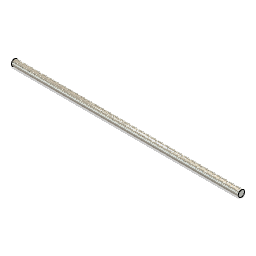
final assembly v7 (Autodesk Fusion 360 archive; units mm, degrees)
design "rod3"
Autodesk Fusion 360 part; units mm, degrees
sketch "Sketch1" plane through (0, 0, 0) normal (1, 0, 0) x (0, 0, -1)
  circle A0 centre (0, 0) radius 3
  dimension "d1" = 6
  constraint coincident A0.centre origin
  measures "d1" diameter of A0
extrude "Extrude1" add sketch "Sketch1" along normal blind 215

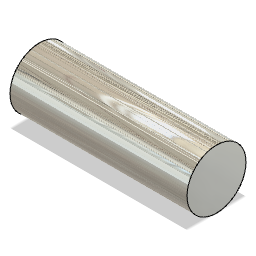
design "rod4"
Autodesk Fusion 360 part; units mm, degrees
sketch "Sketch1" plane through (0, 0, 0) normal (1, 0, 0) x (0, 0, -1)
  circle A0 centre (0, 0) radius 3
  dimension "d1" = 6
  constraint coincident A0.centre origin
  measures "d1" diameter of A0
extrude "Extrude1" add sketch "Sketch1" along normal blind 18

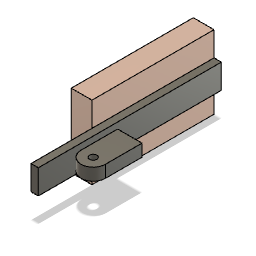
design "stamp pad 1"
Autodesk Fusion 360 part; units mm, degrees
sketch "Sketch1" plane through (0, 0, 0) normal (1, 0, 0) x (0, 0, -1)
  line L0 (-50, 30) -> (50, 30)
  line L1 (50, 30) -> (50, -30)
  line L2 (50, -30) -> (-50, -30)
  line L3 (-50, -30) -> (-50, 30)
  line L4 (48, -28) -> (-48, -28)
  line L5 (-48, -28) -> (-48, 28)
  line L6 (-48, 28) -> (48, 28)
  line L7 (48, 28) -> (48, -28)
  dimension "d1" = 100
  dimension "d2" = 60
  dimension "d3" = 2
  dimension "d17" = 30
  dimension "d18" = 50
  constraint horizontal L0
  constraint perpendicular L0 L1
  constraint parallel L0 L2
  constraint parallel L1 L3
  measures "d1" distance of L1.end L2.end
  measures "d2" distance of L0.end L1.end
  measures "d17" distance of L0 origin
  measures "d18" distance of origin L3
extrude "Extrude1" add sketch "Sketch1" along normal blind 2 contours L0 L1 L2 L3 | L4 L5 L6 L7 makes body 1
extrude "Extrude2" add sketch "Sketch1" against normal blind 15 bodies 1
sketch "Sketch2" plane through (0, 0, 0) normal (-1, 0, 0) x (0, 0, 1)
  line L0 (-48, 28) -> (-48, -28)
  line L1 (-48, -28) -> (48, -28)
  line L2 (48, -28) -> (48, 28)
  line L3 (48, 28) -> (-48, 28)
  line L4 (45, 25) -> (-45, 25)
  line L5 (-45, 25) -> (-45, -25)
  line L6 (-45, -25) -> (45, -25)
  line L7 (45, -25) -> (45, 25)
  line L8 (45, 25) -> (-45, -25) construction
  line L9 (-45, 25) -> (45, -25) construction
  dimension "d8" = 90
  dimension "d9" = 50
  constraint horizontal L4
  constraint perpendicular L4 L5
  constraint parallel L4 L6
  constraint parallel L5 L7
  constraint coincident L8 origin
  constraint coincident L9 origin
  measures "d8" distance of L5.end L6.end
  measures "d9" distance of L4.end L5.end
extrude "Extrude3" add sketch "Sketch2" along normal blind 13 contours L4 L5 L6 L7 bodies 1
sketch "Sketch4" plane through (2, 0, 0) normal (1, 0, 0) x (0, 0, -1)
  line L0 (-50, -30) -> (50, -30)
  line L1 (50, -30) -> (50, 30)
  line L2 (50, 30) -> (-50, 30)
  line L3 (-50, 30) -> (-50, -30)
  line L4 (50, -10) -> (-100, -10)
  line L5 (-100, -10) -> (-100, 10)
  line L6 (-100, 10) -> (50, 10)
  line L7 (50, 10) -> (50, -10)
  point P0 (-50, -10)
  point P1 (50, -10)
  dimension "d22" = 20
  constraint coincident L3 P0
  constraint horizontal L4
  constraint vertical L5
  constraint horizontal L6
  constraint vertical L7
  constraint coincident P1 L4.start
  measures "d22" distance of P1 L6.end
extrude "Extrude4" add sketch "Sketch4" along normal blind 6 contours L3 L4 L5 L6 | L1 L3 L4 L6 L7 bodies 1
sketch "Sketch5" plane through (0, -10, 0) normal (0, -1, 0) x (1, 0, 0)
  line L0 (2, 50) -> (2, -50)
  line L1 (2, -50) -> (8, -50)
  line L2 (8, -50) -> (8, 100)
  line L3 (8, 100) -> (2, 100)
  line L4 (2, 100) -> (2, 50)
  circle A0 centre (18, 65) radius 3
  line L5 (28, 65) -> (28, 35)
  line L6 (28, 35) -> (8, 35)
  arc A1 (28, 65) -> (8, 65) centre (18, 65) ccw
  dimension "d26" = 10
  dimension "d27" = 6
  constraint coincident L2 A1.end
  constraint concentric A0 A1
  constraint tangent L5 A1
  constraint parallel L2 L5
  constraint coincident L2 L6.end
  constraint perpendicular L2 L6
  measures "d26" distance of A1.end A0.centre
  measures "d27" diameter of A0
extrude "Extrude5" add sketch "Sketch5" against normal blind 10 from surface at -5 contours L2 L5 L6 A1 bodies 1
sketch "Sketch6" plane through (0, -30, 0) normal (0, -1, 0) x (1, 0, 0)
  line L0 (-15, -50) -> (2, -50)
  line L1 (2, -50) -> (2, 50)
  line L2 (2, 50) -> (-15, 50)
  line L3 (-15, 50) -> (-15, -50)
  line L4 (-3.4442, -44.9299) -> (-3.4442, 44.3486) construction
  line L5 (-3.4442, 44.3486) -> (-9.7091, 44.3486) construction
  line L6 (-9.7091, 44.3486) -> (-9.7091, -44.9299) construction
  line L7 (-9.7091, -44.9299) -> (-3.4442, -44.9299) construction
  dimension "d32" = 10
  text T0 "STAMP PAD" font "Arial" height 10 align centre middle in box 89.2785 x 6.2649 at (-3.4442, -44.9299) x (0, 1) y (-1, 0) spacing 1 kerned
emboss "Emboss2" depth -2 profiles "Sketch6" section 1 text T0 onto face at (-9.3333, -30, -16.6667) on bodies 1 bodies 1 makes body 2 at (-8.0137, -28, 2.4504) makes body 3 at (-6.6062, -30, 24.3399) makes body 4 at (-8.0137, -30, 15.3972) makes body 5 at (-6.6017, -28, 34.5536) makes body 6 at (-6.6062, -28, -17.8429)

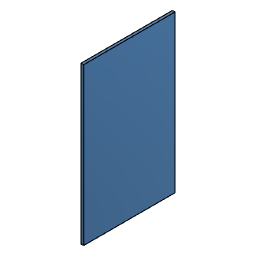
design "base"
Autodesk Fusion 360 part; units mm, degrees
sketch "Sketch1" plane through (0, 0, 0) normal (1, 0, 0) x (0, 0, -1)
  line L0 (0, 0) -> (-350, 0)
  line L1 (-350, 0) -> (-350, 600)
  line L2 (-350, 600) -> (0, 600)
  line L3 (0, 600) -> (0, 0)
  dimension "d1" = 350
  dimension "d2" = 600
  constraint horizontal L0
  constraint vertical L1
  constraint horizontal L2
  constraint vertical L3
  constraint coincident L0.start L3.end
  measures "d1" distance of L0.start L0.end
  measures "d2" distance of L0.start L2.end
extrude "Extrude1" add sketch "Sketch1" along normal blind 10

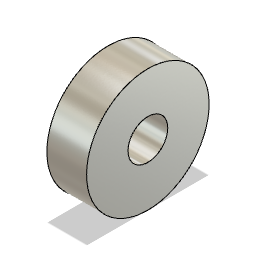
design "bearings"
Autodesk Fusion 360 part; units mm, degrees
sketch "Sketch1" plane through (0, 0, 0) normal (1, 0, 0) x (0, 0, -1)
  circle A0 centre (0, 0) radius 3
  circle A1 centre (0, 0) radius 9.25
  dimension "d1" = 6
  dimension "d2" = 18.5
  constraint coincident A0.centre A1.centre
  constraint concentric A0 A1
  measures "d1" diameter of A0
  measures "d2" diameter of A1
extrude "Extrude1" add sketch "Sketch1" along normal blind 6

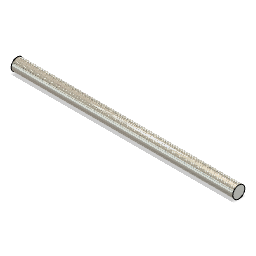
design "rod1"
Autodesk Fusion 360 part; units mm, degrees
sketch "Sketch1" plane through (0, 0, 0) normal (1, 0, 0) x (0, 0, -1)
  circle A0 centre (0, 0) radius 3
  dimension "d1" = 6
  constraint coincident A0.centre origin
  measures "d1" diameter of A0
extrude "Extrude1" add sketch "Sketch1" along normal blind 110

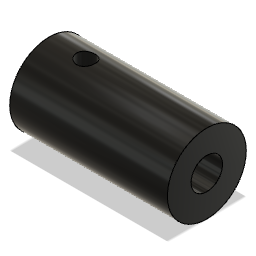
design "motor connector v2"
Autodesk Fusion 360 part; units mm, degrees
sketch "Sketch1" plane through (0, 0, 0) normal (1, 0, 0) x (0, 0, -1)
  circle A0 centre (0, 0) radius 3
  circle A1 centre (0, 0) radius 7.5
  dimension "d1" = 6
  dimension "d2" = 15
  constraint coincident A0.centre A1.centre
  measures "d1" diameter of A0
  measures "d2" diameter of A1
extrude "Extrude1" add sketch "Sketch1" against normal blind 15
sketch "Sketch2" plane through (-15, 0, 0) normal (-1, 0, 0) x (0, 0, 1)
  circle A0 centre (0, 0) radius 7.5
  circle A1 centre (0, 0) radius 3.25
  circle A2 centre (0, 0) radius 7.5
  dimension "d5" = 6.5
  constraint concentric A1 A2
  measures "d5" diameter of A1
extrude "Extrude2" add sketch "Sketch2" along normal blind 15
sketch "Sketch3" plane through (0, 0, 0) normal (0, 1, 0) x (1, 0, 0)
  line L0 (-30, 7.5) -> (-30, -7.5)
  line L1 (0, -7.5) -> (0, 7.5)
  circle A0 centre (-23, 0) radius 1.75
  point P0 (-23, 0)
  dimension "d8" = 30
  constraint coincident P0 A0.centre
  measures "d8" distance of L0 L1
extrude "Extrude3" cut sketch "Sketch3" along normal mid plane 38

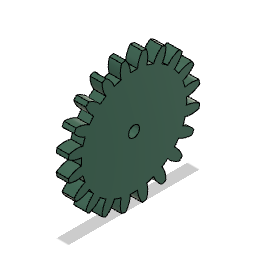
design "6 cm gear"
Autodesk Fusion 360 part; units mm, degrees
sketch "Sketch1" plane through (0, 0, 0) normal (1, 0, 0) x (0, 0, -1)
  arc A0 (28.2536, 4.8202) -> (28.2536, 8.3351) centre (2.0635, 6.5776) ccw
  arc A1 (28.2536, 8.3351) -> (34.8066, 10.6867) centre (27.6511, 20.3199) ccw
  arc A2 (17.9851, 35.4827) -> (16.0896, 36.4485) centre (2.0635, 6.5776) ccw
  arc A3 (8.4852, 32.029) -> (8.2737, 38.988) centre (-3.0992, 35.1595) ccw
  arc A4 (34.8066, 10.6867) -> (34.4738, 12.7878) centre (2.0635, 6.5776) ccw
  arc A5 (6.1726, 39.3208) -> (3.8209, 32.7677) centre (15.8058, 32.1653) ccw
  arc A6 (18.8794, -13.5776) -> (24.6337, -17.4969) centre (28.2213, -6.0457) ccw
  arc A7 (16.0896, -23.2932) -> (17.9851, -22.3274) centre (2.0635, 6.5776) ccw
  arc A8 (22.2187, -10.2383) -> (24.2847, -7.3947) centre (2.0635, 6.5776) ccw
  arc A9 (3.8209, 32.7677) -> (0.306, 32.7677) centre (2.0635, 6.5776) ccw
  arc A10 (0.306, -19.6125) -> (3.8209, -19.6125) centre (2.0635, 6.5776) ccw
  arc A11 (24.6337, -17.4969) -> (26.138, -15.9926) centre (2.0635, 6.5776) ccw
  arc A12 (-13.8582, -22.3274) -> (-11.9627, -23.2932) centre (2.0635, 6.5776) ccw
  arc A13 (31.9343, -7.4485) -> (26.4286, -3.187) centre (22.1521, -14.3991) ccw
  arc A14 (6.1726, 39.3208) -> (3.8209, 32.7677) centre (15.8058, 32.1653) ccw
  arc A15 (-14.7525, -13.5776) -> (-11.9089, -15.6436) centre (2.0635, 6.5776) ccw
  arc A16 (8.2737, -25.8327) -> (8.4852, -18.8737) centre (-3.0992, -22.0043) ccw
  arc A17 (-7.7012, -17.7875) -> (-4.3583, -18.8737) centre (2.0635, 6.5776) ccw
  arc A18 (0.306, -19.6125) -> (3.8209, -19.6125) centre (2.0635, 6.5776) ccw
  arc A19 (26.4286, -3.187) -> (27.5148, 0.1559) centre (2.0635, 6.5776) ccw
  arc A20 (8.4852, -18.8737) -> (11.8281, -17.7875) centre (2.0635, 6.5776) ccw
  arc A21 (8.2737, 38.988) -> (6.1726, 39.3208) centre (2.0635, 6.5776) ccw
  arc A22 (6.1726, -26.1655) -> (8.2737, -25.8327) centre (2.0635, 6.5776) ccw
  arc A23 (8.4852, -18.8737) -> (11.8281, -17.7875) centre (2.0635, 6.5776) ccw
  arc A24 (11.8281, -17.7875) -> (16.0896, -23.2932) centre (23.0402, -13.5111) ccw
  arc A25 (30.9685, -9.344) -> (31.9343, -7.4485) centre (2.0635, 6.5776) ccw
  arc A26 (17.9851, -22.3274) -> (16.0358, -15.6436) centre (5.9857, -22.2007) ccw
  arc A27 (6.1726, -26.1655) -> (8.2737, -25.8327) centre (2.0635, 6.5776) ccw
  arc A28 (3.8209, -19.6125) -> (6.1726, -26.1655) centre (15.8058, -19.01) ccw
  arc A29 (34.4738, 0.3674) -> (34.8066, 2.4685) centre (2.0635, 6.5776) ccw
  arc A30 (34.8066, 2.4685) -> (28.2536, 4.8202) centre (27.6511, -7.1647) ccw
  arc A31 (18.8794, 26.7329) -> (16.0358, 28.7989) centre (2.0635, 6.5776) ccw
  arc A32 (-11.9089, -15.6436) -> (-13.8582, -22.3274) centre (-1.8588, -22.2007) ccw
  arc A33 (11.8281, -17.7875) -> (16.0896, -23.2932) centre (23.0402, -13.5111) ccw
  arc A34 (8.4852, 32.029) -> (8.2737, 38.988) centre (-3.0992, 35.1595) ccw
  arc A35 (16.0896, -23.2932) -> (17.9851, -22.3274) centre (2.0635, 6.5776) ccw
  arc A36 (16.0896, 36.4485) -> (11.8281, 30.9428) centre (23.0402, 26.6663) ccw
  arc A37 (16.0358, -15.6436) -> (18.8794, -13.5776) centre (2.0635, 6.5776) ccw
  arc A38 (-4.3583, -18.8737) -> (-4.1467, -25.8327) centre (7.2261, -22.0043) ccw
  arc A39 (-11.9627, -23.2932) -> (-7.7012, -17.7875) centre (-18.9133, -13.5111) ccw
  arc A40 (3.8209, -19.6125) -> (6.1726, -26.1655) centre (15.8058, -19.01) ccw
  arc A41 (11.8281, 30.9428) -> (8.4852, 32.029) centre (2.0635, 6.5776) ccw
  arc A42 (-4.1467, -25.8327) -> (-2.0457, -26.1655) centre (2.0635, 6.5776) ccw
  arc A43 (17.9851, -22.3274) -> (16.0358, -15.6436) centre (5.9857, -22.2007) ccw
  arc A44 (16.0358, -15.6436) -> (18.8794, -13.5776) centre (2.0635, 6.5776) ccw
  arc A45 (24.2847, -7.3947) -> (30.9685, -9.344) centre (30.8418, 2.6554) ccw
  arc A46 (30.9685, 22.4993) -> (24.2847, 20.55) centre (30.8418, 10.4999) ccw
  arc A47 (18.8794, 26.7329) -> (16.0358, 28.7989) centre (2.0635, 6.5776) ccw
  arc A48 (26.138, 29.1479) -> (24.6337, 30.6521) centre (2.0635, 6.5776) ccw
  arc A49 (24.2847, 20.55) -> (22.2187, 23.3936) centre (2.0635, 6.5776) ccw
  arc A50 (27.5148, 12.9994) -> (26.4286, 16.3423) centre (2.0635, 6.5776) ccw
  arc A51 (17.9851, 35.4827) -> (16.0896, 36.4485) centre (2.0635, 6.5776) ccw
  arc A52 (31.9343, 20.6038) -> (30.9685, 22.4993) centre (2.0635, 6.5776) ccw
  arc A53 (8.2737, 38.988) -> (6.1726, 39.3208) centre (2.0635, 6.5776) ccw
  arc A54 (16.0896, 36.4485) -> (11.8281, 30.9428) centre (23.0402, 26.6663) ccw
  arc A55 (24.6337, 30.6521) -> (18.8794, 26.7329) centre (28.2213, 19.201) ccw
  arc A56 (16.0358, 28.7989) -> (17.9851, 35.4827) centre (5.9857, 35.356) ccw
  arc A57 (-2.0457, -26.1655) -> (0.306, -19.6125) centre (-11.6789, -19.01) ccw
  arc A58 (16.0358, 28.7989) -> (17.9851, 35.4827) centre (5.9857, 35.356) ccw
  arc A59 (27.5148, 0.1559) -> (34.4738, 0.3674) centre (30.6454, 11.7403) ccw
  arc A60 (8.2737, -25.8327) -> (8.4852, -18.8737) centre (-3.0992, -22.0043) ccw
  arc A61 (3.8209, 32.7677) -> (0.306, 32.7677) centre (2.0635, 6.5776) ccw
  arc A62 (26.4286, 16.3423) -> (31.9343, 20.6038) centre (22.1521, 27.5544) ccw
  arc A63 (22.2187, 23.3936) -> (26.138, 29.1479) centre (14.6868, 32.7354) ccw
  arc A64 (11.8281, 30.9428) -> (8.4852, 32.029) centre (2.0635, 6.5776) ccw
  arc A65 (34.4738, 12.7878) -> (27.5148, 12.9994) centre (30.6454, 1.4149) ccw
  arc A66 (-27.8074, -7.4485) -> (-26.8416, -9.344) centre (2.0635, 6.5776) ccw
  arc A67 (30.9685, 22.4993) -> (24.2847, 20.55) centre (30.8418, 10.4999) ccw
  arc A68 (-14.7525, -13.5776) -> (-11.9089, -15.6436) centre (2.0635, 6.5776) ccw
  arc A69 (-7.7012, -17.7875) -> (-4.3583, -18.8737) centre (2.0635, 6.5776) ccw
  arc A70 (-4.3583, -18.8737) -> (-4.1467, -25.8327) centre (7.2261, -22.0043) ccw
  arc A71 (-20.5068, -17.4969) -> (-14.7525, -13.5776) centre (-24.0944, -6.0457) ccw
  arc A72 (-13.8582, -22.3274) -> (-11.9627, -23.2932) centre (2.0635, 6.5776) ccw
  arc A73 (-18.0918, -10.2383) -> (-22.0111, -15.9926) centre (-10.5599, -19.5802) ccw
  arc A74 (-30.6797, 2.4685) -> (-30.3469, 0.3674) centre (2.0635, 6.5776) ccw
  arc A75 (-27.8074, 20.6038) -> (-22.3017, 16.3423) centre (-18.0252, 27.5544) ccw
  arc A76 (-11.9089, 28.7989) -> (-14.7525, 26.7329) centre (2.0635, 6.5776) ccw
  arc A77 (24.6337, 30.6521) -> (18.8794, 26.7329) centre (28.2213, 19.201) ccw
  arc A78 (-18.0918, 23.3936) -> (-20.1578, 20.55) centre (2.0635, 6.5776) ccw
  arc A79 (-30.3469, 0.3674) -> (-23.3879, 0.1559) centre (-26.5185, 11.7403) ccw
  arc A80 (34.4738, 0.3674) -> (34.8066, 2.4685) centre (2.0635, 6.5776) ccw
  arc A81 (-7.7012, 30.9428) -> (-11.9627, 36.4485) centre (-18.9133, 26.6663) ccw
  arc A82 (34.8066, 2.4685) -> (28.2536, 4.8202) centre (27.6511, -7.1647) ccw
  arc A83 (-4.1467, 38.988) -> (-4.3583, 32.029) centre (7.2261, 35.1595) ccw
  arc A84 (-18.0918, -10.2383) -> (-22.0111, -15.9926) centre (-10.5599, -19.5802) ccw
  arc A85 (26.138, 29.1479) -> (24.6337, 30.6521) centre (2.0635, 6.5776) ccw
  arc A86 (-22.0111, -15.9926) -> (-20.5068, -17.4969) centre (2.0635, 6.5776) ccw
  arc A87 (-20.1578, -7.3947) -> (-18.0918, -10.2383) centre (2.0635, 6.5776) ccw
  arc A88 (-24.1266, 8.3351) -> (-24.1266, 4.8202) centre (2.0635, 6.5776) ccw
  arc A89 (-26.8416, -9.344) -> (-20.1578, -7.3947) centre (-26.7149, 2.6554) ccw
  arc A90 (22.2187, 23.3936) -> (26.138, 29.1479) centre (14.6868, 32.7354) ccw
  arc A91 (28.2536, 4.8202) -> (28.2536, 8.3351) centre (2.0635, 6.5776) ccw
  arc A92 (24.6337, -17.4969) -> (26.138, -15.9926) centre (2.0635, 6.5776) ccw
  arc A93 (-27.8074, -7.4485) -> (-26.8416, -9.344) centre (2.0635, 6.5776) ccw
  arc A94 (22.2187, -10.2383) -> (24.2847, -7.3947) centre (2.0635, 6.5776) ccw
  arc A95 (34.8066, 10.6867) -> (34.4738, 12.7878) centre (2.0635, 6.5776) ccw
  arc A96 (27.5148, 12.9994) -> (26.4286, 16.3423) centre (2.0635, 6.5776) ccw
  arc A97 (24.2847, 20.55) -> (22.2187, 23.3936) centre (2.0635, 6.5776) ccw
  arc A98 (28.2536, 8.3351) -> (34.8066, 10.6867) centre (27.6511, 20.3199) ccw
  arc A99 (-26.8416, 22.4993) -> (-27.8074, 20.6038) centre (2.0635, 6.5776) ccw
  arc A100 (-11.9627, -23.2932) -> (-7.7012, -17.7875) centre (-18.9133, -13.5111) ccw
  arc A101 (27.5148, 0.1559) -> (34.4738, 0.3674) centre (30.6454, 11.7403) ccw
  arc A102 (34.4738, 12.7878) -> (27.5148, 12.9994) centre (30.6454, 1.4149) ccw
  arc A103 (-22.3017, -3.187) -> (-27.8074, -7.4485) centre (-18.0252, -14.3991) ccw
  arc A104 (-20.5068, 30.6521) -> (-22.0111, 29.1479) centre (2.0635, 6.5776) ccw
  arc A105 (26.138, -15.9926) -> (22.2187, -10.2383) centre (14.6868, -19.5802) ccw
  arc A106 (26.4286, -3.187) -> (27.5148, 0.1559) centre (2.0635, 6.5776) ccw
  arc A107 (18.8794, -13.5776) -> (24.6337, -17.4969) centre (28.2213, -6.0457) ccw
  arc A108 (30.9685, -9.344) -> (31.9343, -7.4485) centre (2.0635, 6.5776) ccw
  arc A109 (31.9343, -7.4485) -> (26.4286, -3.187) centre (22.1521, -14.3991) ccw
  arc A110 (-23.3879, 0.1559) -> (-22.3017, -3.187) centre (2.0635, 6.5776) ccw
  arc A111 (26.4286, 16.3423) -> (31.9343, 20.6038) centre (22.1521, 27.5544) ccw
  arc A112 (31.9343, 20.6038) -> (30.9685, 22.4993) centre (2.0635, 6.5776) ccw
  arc A113 (-30.3469, 0.3674) -> (-23.3879, 0.1559) centre (-26.5185, 11.7403) ccw
  arc A114 (24.2847, -7.3947) -> (30.9685, -9.344) centre (30.8418, 2.6554) ccw
  arc A115 (-14.7525, 26.7329) -> (-20.5068, 30.6521) centre (-24.0944, 19.201) ccw
  arc A116 (-26.8416, -9.344) -> (-20.1578, -7.3947) centre (-26.7149, 2.6554) ccw
  arc A117 (-20.1578, -7.3947) -> (-18.0918, -10.2383) centre (2.0635, 6.5776) ccw
  arc A118 (0.306, 32.7677) -> (-2.0457, 39.3208) centre (-11.6789, 32.1653) ccw
  arc A119 (-24.1266, 4.8202) -> (-30.6797, 2.4685) centre (-23.5242, -7.1647) ccw
  arc A120 (-26.8416, 22.4993) -> (-27.8074, 20.6038) centre (2.0635, 6.5776) ccw
  arc A121 (-30.3469, 12.7878) -> (-30.6797, 10.6867) centre (2.0635, 6.5776) ccw
  arc A122 (-11.9089, -15.6436) -> (-13.8582, -22.3274) centre (-1.8588, -22.2007) ccw
  arc A123 (-4.1467, -25.8327) -> (-2.0457, -26.1655) centre (2.0635, 6.5776) ccw
  arc A124 (-23.3879, 12.9994) -> (-30.3469, 12.7878) centre (-26.5185, 1.4149) ccw
  arc A125 (-22.0111, 29.1479) -> (-18.0918, 23.3936) centre (-10.5599, 32.7354) ccw
  arc A126 (-22.3017, -3.187) -> (-27.8074, -7.4485) centre (-18.0252, -14.3991) ccw
  arc A127 (-20.5068, -17.4969) -> (-14.7525, -13.5776) centre (-24.0944, -6.0457) ccw
  arc A128 (-4.3583, 32.029) -> (-7.7012, 30.9428) centre (2.0635, 6.5776) ccw
  arc A129 (-2.0457, 39.3208) -> (-4.1467, 38.988) centre (2.0635, 6.5776) ccw
  arc A130 (-18.0918, 23.3936) -> (-20.1578, 20.55) centre (2.0635, 6.5776) ccw
  arc A131 (-23.3879, 0.1559) -> (-22.3017, -3.187) centre (2.0635, 6.5776) ccw
  arc A132 (-20.1578, 20.55) -> (-26.8416, 22.4993) centre (-26.7149, 10.4999) ccw
  arc A133 (-27.8074, 20.6038) -> (-22.3017, 16.3423) centre (-18.0252, 27.5544) ccw
  arc A134 (-2.0457, -26.1655) -> (0.306, -19.6125) centre (-11.6789, -19.01) ccw
  arc A135 (-22.0111, -15.9926) -> (-20.5068, -17.4969) centre (2.0635, 6.5776) ccw
  arc A136 (-24.1266, 8.3351) -> (-24.1266, 4.8202) centre (2.0635, 6.5776) ccw
  arc A137 (-24.1266, 4.8202) -> (-30.6797, 2.4685) centre (-23.5242, -7.1647) ccw
  arc A138 (-14.7525, 26.7329) -> (-20.5068, 30.6521) centre (-24.0944, 19.201) ccw
  arc A139 (-11.9627, 36.4485) -> (-13.8582, 35.4827) centre (2.0635, 6.5776) ccw
  arc A140 (-2.0457, 39.3208) -> (-4.1467, 38.988) centre (2.0635, 6.5776) ccw
  arc A141 (-20.1578, 20.55) -> (-26.8416, 22.4993) centre (-26.7149, 10.4999) ccw
  arc A142 (-30.3469, 12.7878) -> (-30.6797, 10.6867) centre (2.0635, 6.5776) ccw
  arc A143 (-20.5068, 30.6521) -> (-22.0111, 29.1479) centre (2.0635, 6.5776) ccw
  arc A144 (-4.1467, 38.988) -> (-4.3583, 32.029) centre (7.2261, 35.1595) ccw
  arc A145 (-11.9627, 36.4485) -> (-13.8582, 35.4827) centre (2.0635, 6.5776) ccw
  arc A146 (-30.6797, 2.4685) -> (-30.3469, 0.3674) centre (2.0635, 6.5776) ccw
  arc A147 (0.306, 32.7677) -> (-2.0457, 39.3208) centre (-11.6789, 32.1653) ccw
  arc A148 (-23.3879, 12.9994) -> (-30.3469, 12.7878) centre (-26.5185, 1.4149) ccw
  arc A149 (-13.8582, 35.4827) -> (-11.9089, 28.7989) centre (-1.8588, 35.356) ccw
  arc A150 (-13.8582, 35.4827) -> (-11.9089, 28.7989) centre (-1.8588, 35.356) ccw
  arc A151 (-22.3017, 16.3423) -> (-23.3879, 12.9994) centre (2.0635, 6.5776) ccw
  arc A152 (-4.3583, 32.029) -> (-7.7012, 30.9428) centre (2.0635, 6.5776) ccw
  arc A153 (-11.9089, 28.7989) -> (-14.7525, 26.7329) centre (2.0635, 6.5776) ccw
  arc A154 (-22.3017, 16.3423) -> (-23.3879, 12.9994) centre (2.0635, 6.5776) ccw
  arc A155 (-22.0111, 29.1479) -> (-18.0918, 23.3936) centre (-10.5599, 32.7354) ccw
  arc A156 (-7.7012, 30.9428) -> (-11.9627, 36.4485) centre (-18.9133, 26.6663) ccw
  arc A157 (-30.6797, 10.6867) -> (-24.1266, 8.3351) centre (-23.5242, 20.3199) ccw
  arc A158 (-30.6797, 10.6867) -> (-24.1266, 8.3351) centre (-23.5242, 20.3199) ccw
  arc A159 (26.138, -15.9926) -> (22.2187, -10.2383) centre (14.6868, -19.5802) ccw
  circle A160 centre (2.0635, 6.5776) radius 2.75
  dimension "d4" = 5.5
  constraint concentric A88 A160
  measures "d4" diameter of A160
extrude "Extrude1" add sketch "Sketch1" along normal blind 6

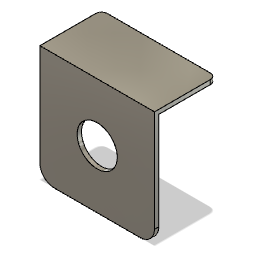
design "Motor clamp"
Autodesk Fusion 360 part; units mm, degrees
sketch "Sketch1" plane through (0, 0, 0) normal (0, 1, 0) x (1, 0, 0)
  line L0 (18, 10.75) -> (-18, 10.75)
  line L1 (-20, 8.75) -> (-20, -10.75)
  line L2 (-20, -10.75) -> (20, -10.75)
  line L3 (20, -10.75) -> (20, 8.75)
  line L4 (20, 10.75) -> (-20, -10.75) construction
  line L5 (-20, 10.75) -> (20, -10.75) construction
  arc A0 (-18, 10.75) -> (-20, 8.75) centre (-18, 8.75) ccw
  arc A1 (20, 8.75) -> (18, 10.75) centre (18, 8.75) ccw
  dimension "d1" = 40
  dimension "d2" = 21.5
  dimension "d3" = 2
  constraint horizontal L0
  constraint perpendicular L0 L1
  constraint parallel L0 L2
  constraint parallel L1 L3
  constraint coincident L4 origin
  constraint coincident L5 origin
  constraint coincident L5.start L0
  constraint coincident L5.start L1
  constraint tangent L0 A0
  constraint tangent L1 A0
  constraint coincident L4.start L0
  constraint coincident L4.start L3
  constraint tangent L0 A1
  constraint tangent L3 A1
  constraint equal A0 A1
  measures "d1" distance of L1.end L2.end
  measures "d2" distance of L5.start L1.end
  measures "d3" radius of A0
extrude "Extrude1" add sketch "Sketch1" along normal blind 1.5
sketch "Sketch2" plane through (0, 0, 10.75) normal (0, 0, 1) x (1, 0, 0)
  line L0 (-20, 0) -> (20, 0)
  line L1 (20, 0) -> (20, 1.5)
  line L2 (20, 1.5) -> (-20, 1.5)
  line L3 (-20, 1.5) -> (-20, 0)
  line L4 (-20, 1.5) -> (20, 1.5)
  line L5 (20, 1.5) -> (20, -34)
  line L6 (15, -39) -> (-15, -39)
  line L7 (-20, -34) -> (-20, 1.5)
  circle A0 centre (0, -18.75) radius 7
  arc A1 (-20, -34) -> (-15, -39) centre (-15, -34) ccw
  arc A2 (15, -39) -> (20, -34) centre (15, -34) ccw
  point P0 (-20, -39)
  dimension "d7" = 40.5
  dimension "d8" = 14
  dimension "d11" = 5
  constraint horizontal L4
  constraint vertical L5
  constraint horizontal L6
  constraint vertical L7
  constraint coincident L2.end L3.start
  constraint coincident P0 L7
  constraint coincident P0 L6
  constraint tangent L7 A1
  constraint tangent L6 A1
  constraint tangent L5 A2
  constraint tangent L6 A2
  constraint equal A1 A2
  measures "d7" distance of L2.end P0
  measures "d8" diameter of A0
  measures "d11" radius of A1
extrude "Extrude2" add sketch "Sketch2" against normal blind 1.5

design "Coupler_B"
Autodesk Fusion 360 part; units mm, degrees
sketch "Sketch1" plane through (0, 0, 0) normal (0, 1, 0) x (1, 0, 0)
  line L0 (-12.5, -96.75) -> (-12.5, 96.75)
  line L1 (12.5, 96.75) -> (12.5, -96.75)
  circle A0 centre (0, -96.75) radius 9.25
  arc A1 (-12.5, -96.75) -> (12.5, -96.75) centre (0, -96.75) ccw
  circle A2 centre (0, 96.75) radius 9.25
  arc A3 (12.5, 96.75) -> (-12.5, 96.75) centre (0, 96.75) ccw
  constraint parallel L0 L1
  constraint concentric A0 A1
extrude "Extrude1" add sketch "Sketch1" along normal blind 6

design "4 cm gear"
Autodesk Fusion 360 part; units mm, degrees
sketch "Sketch1" plane through (0, 0, 0) normal (1, 0, 0) x (0, 0, -1)
  arc A0 (30.8871, 27.0565) -> (30.1313, 27.8123) centre (14.9574, 11.8827) ccw
  arc A1 (10.989, -9.7564) -> (12.0447, -9.9237) centre (14.9574, 11.8827) ccw
  arc A2 (4.4964, -7.4711) -> (5.4488, -7.9563) centre (14.9574, 11.8827) ccw
  arc A3 (12.0447, 33.689) -> (10.989, 33.5218) centre (14.9574, 11.8827) ccw
  arc A4 (24.4289, 26.5968) -> (25.4184, 31.2364) centre (17.4515, 30.5103) ccw
  arc A5 (34.3112, 22.3437) -> (29.6716, 21.3542) centre (33.5851, 14.3767) ccw
  arc A6 (25.4184, -7.4711) -> (24.4289, -2.8315) centre (17.4515, -6.745) ccw
  arc A7 (32.4286, 10.8965) -> (32.4286, 12.8689) centre (14.9574, 11.8827) ccw
  arc A8 (36.5965, 7.9143) -> (36.7638, 8.97) centre (14.9574, 11.8827) ccw
  arc A9 (30.8871, -3.2912) -> (28.5123, 0.8155) centre (23.0856, -5.0625) ccw
  arc A10 (1.4026, 0.8155) -> (-0.9722, -3.2912) centre (6.8292, -5.0625) ccw
  arc A11 (-1.3539, 18.2195) -> (-1.9634, 16.3437) centre (14.9574, 11.8827) ccw
  arc A12 (-2.5138, 12.8689) -> (-2.5138, 10.8965) centre (14.9574, 11.8827) ccw
  arc A13 (-1.9634, 16.3437) -> (-6.6817, 15.8511) centre (-3.5292, 8.4984) ccw
  arc A14 (28.5123, 0.8155) -> (29.6716, 2.4112) centre (14.9574, 11.8827) ccw
  arc A15 (10.989, -9.7564) -> (12.0447, -9.9237) centre (14.9574, 11.8827) ccw
  arc A16 (29.6716, 2.4112) -> (34.3112, 1.4217) centre (33.5851, 9.3886) ccw
  arc A17 (8.6206, -4.4287) -> (10.4964, -5.0382) centre (14.9574, 11.8827) ccw
  arc A18 (36.7638, 8.97) -> (32.4286, 10.8965) centre (31.4935, 2.9514) ccw
  arc A19 (28.5123, 0.8155) -> (29.6716, 2.4112) centre (14.9574, 11.8827) ccw
  arc A20 (5.4859, -2.8315) -> (4.4964, -7.4711) centre (12.4634, -6.745) ccw
  arc A21 (24.4661, 31.7217) -> (21.2942, 28.194) centre (28.5615, 24.8494) ccw
  arc A22 (-0.9722, 27.0565) -> (1.4026, 22.9498) centre (6.8292, 28.8279) ccw
  arc A23 (21.2942, -4.4287) -> (24.4661, -7.9563) centre (28.5615, -1.0841) ccw
  arc A24 (25.4184, 31.2364) -> (24.4661, 31.7217) centre (14.9574, 11.8827) ccw
  arc A25 (-1.3539, 5.5459) -> (-4.8816, 2.374) centre (1.9907, -1.7214) ccw
  arc A26 (25.4184, -7.4711) -> (24.4289, -2.8315) centre (17.4515, -6.745) ccw
  arc A27 (5.4859, 26.5968) -> (3.8903, 25.4375) centre (14.9574, 11.8827) ccw
  arc A28 (-0.9722, -3.2912) -> (-0.2164, -4.047) centre (14.9574, 11.8827) ccw
  arc A29 (-6.8489, 8.97) -> (-6.6817, 7.9143) centre (14.9574, 11.8827) ccw
  arc A30 (24.4661, -7.9563) -> (25.4184, -7.4711) centre (14.9574, 11.8827) ccw
  arc A31 (10.989, 33.5218) -> (10.4964, 28.8035) centre (18.3417, 30.3693) ccw
  arc A32 (-0.2164, -4.047) -> (3.8903, -1.6722) centre (-1.9878, 3.7545) ccw
  arc A33 (18.9258, 33.5218) -> (17.8701, 33.689) centre (14.9574, 11.8827) ccw
  arc A34 (3.8903, 25.4375) -> (-0.2164, 27.8123) centre (-1.9878, 20.0109) ccw
  arc A35 (12.0447, 33.689) -> (10.989, 33.5218) centre (14.9574, 11.8827) ccw
  arc A36 (0.2433, 2.4112) -> (1.4026, 0.8155) centre (14.9574, 11.8827) ccw
  arc A37 (-0.9722, 27.0565) -> (1.4026, 22.9498) centre (6.8292, 28.8279) ccw
  arc A38 (24.4289, -2.8315) -> (26.0246, -1.6722) centre (14.9574, 11.8827) ccw
  arc A39 (-6.8489, 8.97) -> (-6.6817, 7.9143) centre (14.9574, 11.8827) ccw
  arc A40 (-4.3963, 1.4217) -> (0.2433, 2.4112) centre (-3.6702, 9.3886) ccw
  arc A41 (1.4026, 0.8155) -> (-0.9722, -3.2912) centre (6.8292, -5.0625) ccw
  arc A42 (-0.2164, 27.8123) -> (-0.9722, 27.0565) centre (14.9574, 11.8827) ccw
  arc A43 (8.6206, 28.194) -> (5.4488, 31.7217) centre (1.3533, 24.8494) ccw
  arc A44 (4.4964, 31.2364) -> (5.4859, 26.5968) centre (12.4634, 30.5103) ccw
  arc A45 (0.2433, 21.3542) -> (-4.3963, 22.3437) centre (-3.6702, 14.3767) ccw
  arc A46 (18.9258, 33.5218) -> (17.8701, 33.689) centre (14.9574, 11.8827) ccw
  arc A47 (4.4964, 31.2364) -> (5.4859, 26.5968) centre (12.4634, 30.5103) ccw
  arc A48 (19.4184, 28.8035) -> (18.9258, 33.5218) centre (11.5731, 30.3693) ccw
  arc A49 (-1.9634, 7.4217) -> (-1.3539, 5.5459) centre (14.9574, 11.8827) ccw
  arc A50 (10.4964, -5.0382) -> (10.989, -9.7564) centre (18.3417, -6.604) ccw
  arc A51 (30.8871, 27.0565) -> (30.1313, 27.8123) centre (14.9574, 11.8827) ccw
  arc A52 (-4.8816, 2.374) -> (-4.3963, 1.4217) centre (14.9574, 11.8827) ccw
  arc A53 (21.2942, 28.194) -> (19.4184, 28.8035) centre (14.9574, 11.8827) ccw
  arc A54 (-0.9722, -3.2912) -> (-0.2164, -4.047) centre (14.9574, 11.8827) ccw
  arc A55 (30.1313, 27.8123) -> (26.0246, 25.4375) centre (31.9027, 20.0109) ccw
  arc A56 (-4.3963, 22.3437) -> (-4.8816, 21.3913) centre (14.9574, 11.8827) ccw
  arc A57 (13.9712, 29.3539) -> (12.0447, 33.689) centre (6.0261, 28.4187) ccw
  arc A58 (-2.5138, 10.8965) -> (-6.8489, 8.97) centre (-1.5786, 2.9514) ccw
  arc A59 (13.9712, 29.3539) -> (12.0447, 33.689) centre (6.0261, 28.4187) ccw
  arc A60 (34.7964, 21.3913) -> (34.3112, 22.3437) centre (14.9574, 11.8827) ccw
  arc A61 (8.6206, 28.194) -> (5.4488, 31.7217) centre (1.3533, 24.8494) ccw
  arc A62 (-2.5138, 12.8689) -> (-2.5138, 10.8965) centre (14.9574, 11.8827) ccw
  arc A63 (19.4184, -5.0382) -> (21.2942, -4.4287) centre (14.9574, 11.8827) ccw
  arc A64 (13.9712, -5.5885) -> (15.9436, -5.5885) centre (14.9574, 11.8827) ccw
  arc A65 (30.1313, 27.8123) -> (26.0246, 25.4375) centre (31.9027, 20.0109) ccw
  arc A66 (19.4184, 28.8035) -> (18.9258, 33.5218) centre (11.5731, 30.3693) ccw
  arc A67 (18.9258, -9.7564) -> (19.4184, -5.0382) centre (11.5731, -6.604) ccw
  arc A68 (-6.6817, 7.9143) -> (-1.9634, 7.4217) centre (-3.5292, 15.267) ccw
  arc A69 (5.4488, 31.7217) -> (4.4964, 31.2364) centre (14.9574, 11.8827) ccw
  arc A70 (12.0447, -9.9237) -> (13.9712, -5.5885) centre (6.0261, -4.6534) ccw
  arc A71 (36.7638, 14.7954) -> (36.5965, 15.8511) centre (14.9574, 11.8827) ccw
  arc A72 (32.4286, 12.8689) -> (36.7638, 14.7954) centre (31.4935, 20.814) ccw
  arc A73 (10.4964, 28.8035) -> (8.6206, 28.194) centre (14.9574, 11.8827) ccw
  arc A74 (15.9436, -5.5885) -> (17.8701, -9.9237) centre (23.8887, -4.6534) ccw
  arc A75 (17.8701, -9.9237) -> (18.9258, -9.7564) centre (14.9574, 11.8827) ccw
  arc A76 (1.4026, 22.9498) -> (0.2433, 21.3542) centre (14.9574, 11.8827) ccw
  arc A77 (26.0246, 25.4375) -> (24.4289, 26.5968) centre (14.9574, 11.8827) ccw
  arc A78 (17.8701, 33.689) -> (15.9436, 29.3539) centre (23.8887, 28.4187) ccw
  arc A79 (32.4286, 10.8965) -> (32.4286, 12.8689) centre (14.9574, 11.8827) ccw
  arc A80 (15.9436, 29.3539) -> (13.9712, 29.3539) centre (14.9574, 11.8827) ccw
  arc A81 (24.4289, 26.5968) -> (25.4184, 31.2364) centre (17.4515, 30.5103) ccw
  arc A82 (32.4286, 12.8689) -> (36.7638, 14.7954) centre (31.4935, 20.814) ccw
  arc A83 (25.4184, 31.2364) -> (24.4661, 31.7217) centre (14.9574, 11.8827) ccw
  arc A84 (36.7638, 14.7954) -> (36.5965, 15.8511) centre (14.9574, 11.8827) ccw
  arc A85 (34.7964, 21.3913) -> (34.3112, 22.3437) centre (14.9574, 11.8827) ccw
  arc A86 (31.2688, 18.2195) -> (34.7964, 21.3913) centre (27.9242, 25.4868) ccw
  arc A87 (28.5123, 22.9498) -> (30.8871, 27.0565) centre (23.0856, 28.8279) ccw
  arc A88 (34.3112, 22.3437) -> (29.6716, 21.3542) centre (33.5851, 14.3767) ccw
  arc A89 (31.8783, 16.3437) -> (31.2688, 18.2195) centre (14.9574, 11.8827) ccw
  arc A90 (36.5965, 15.8511) -> (31.8783, 16.3437) centre (33.4441, 8.4984) ccw
  arc A91 (29.6716, 21.3542) -> (28.5123, 22.9498) centre (14.9574, 11.8827) ccw
  arc A92 (-4.8816, 21.3913) -> (-1.3539, 18.2195) centre (1.9907, 25.4868) ccw
  arc A93 (4.4964, -7.4711) -> (5.4488, -7.9563) centre (14.9574, 11.8827) ccw
  arc A94 (30.1313, -4.047) -> (30.8871, -3.2912) centre (14.9574, 11.8827) ccw
  arc A95 (5.4859, -2.8315) -> (4.4964, -7.4711) centre (12.4634, -6.745) ccw
  arc A96 (5.4488, -7.9563) -> (8.6206, -4.4287) centre (1.3533, -1.0841) ccw
  arc A97 (26.0246, -1.6722) -> (30.1313, -4.047) centre (31.9027, 3.7545) ccw
  arc A98 (-1.3539, 18.2195) -> (-1.9634, 16.3437) centre (14.9574, 11.8827) ccw
  arc A99 (10.989, 33.5218) -> (10.4964, 28.8035) centre (18.3417, 30.3693) ccw
  arc A100 (30.1313, -4.047) -> (30.8871, -3.2912) centre (14.9574, 11.8827) ccw
  arc A101 (-4.3963, 22.3437) -> (-4.8816, 21.3913) centre (14.9574, 11.8827) ccw
  arc A102 (21.2942, -4.4287) -> (24.4661, -7.9563) centre (28.5615, -1.0841) ccw
  arc A103 (15.9436, -5.5885) -> (17.8701, -9.9237) centre (23.8887, -4.6534) ccw
  arc A104 (29.6716, 2.4112) -> (34.3112, 1.4217) centre (33.5851, 9.3886) ccw
  arc A105 (18.9258, -9.7564) -> (19.4184, -5.0382) centre (11.5731, -6.604) ccw
  arc A106 (3.8903, -1.6722) -> (5.4859, -2.8315) centre (14.9574, 11.8827) ccw
  arc A107 (31.8783, 7.4217) -> (36.5965, 7.9143) centre (33.4441, 15.267) ccw
  arc A108 (34.3112, 1.4217) -> (34.7964, 2.374) centre (14.9574, 11.8827) ccw
  arc A109 (1.4026, 22.9498) -> (0.2433, 21.3542) centre (14.9574, 11.8827) ccw
  arc A110 (0.2433, 21.3542) -> (-4.3963, 22.3437) centre (-3.6702, 14.3767) ccw
  arc A111 (34.7964, 2.374) -> (31.2688, 5.5459) centre (27.9242, -1.7214) ccw
  arc A112 (24.4661, -7.9563) -> (25.4184, -7.4711) centre (14.9574, 11.8827) ccw
  arc A113 (26.0246, -1.6722) -> (30.1313, -4.047) centre (31.9027, 3.7545) ccw
  arc A114 (31.2688, 5.5459) -> (31.8783, 7.4217) centre (14.9574, 11.8827) ccw
  arc A115 (10.4964, -5.0382) -> (10.989, -9.7564) centre (18.3417, -6.604) ccw
  arc A116 (12.0447, -9.9237) -> (13.9712, -5.5885) centre (6.0261, -4.6534) ccw
  arc A117 (-6.6817, 15.8511) -> (-6.8489, 14.7954) centre (14.9574, 11.8827) ccw
  arc A118 (34.3112, 1.4217) -> (34.7964, 2.374) centre (14.9574, 11.8827) ccw
  arc A119 (24.4289, -2.8315) -> (26.0246, -1.6722) centre (14.9574, 11.8827) ccw
  arc A120 (-6.8489, 14.7954) -> (-2.5138, 12.8689) centre (-1.5786, 20.814) ccw
  arc A121 (-4.8816, 2.374) -> (-4.3963, 1.4217) centre (14.9574, 11.8827) ccw
  arc A122 (10.4964, 28.8035) -> (8.6206, 28.194) centre (14.9574, 11.8827) ccw
  arc A123 (5.4859, 26.5968) -> (3.8903, 25.4375) centre (14.9574, 11.8827) ccw
  arc A124 (36.5965, 7.9143) -> (36.7638, 8.97) centre (14.9574, 11.8827) ccw
  arc A125 (3.8903, -1.6722) -> (5.4859, -2.8315) centre (14.9574, 11.8827) ccw
  arc A126 (-2.5138, 10.8965) -> (-6.8489, 8.97) centre (-1.5786, 2.9514) ccw
  arc A127 (5.4488, 31.7217) -> (4.4964, 31.2364) centre (14.9574, 11.8827) ccw
  arc A128 (-4.3963, 1.4217) -> (0.2433, 2.4112) centre (-3.6702, 9.3886) ccw
  arc A129 (34.7964, 2.374) -> (31.2688, 5.5459) centre (27.9242, -1.7214) ccw
  arc A130 (13.9712, -5.5885) -> (15.9436, -5.5885) centre (14.9574, 11.8827) ccw
  arc A131 (-6.6817, 7.9143) -> (-1.9634, 7.4217) centre (-3.5292, 15.267) ccw
  arc A132 (31.8783, 7.4217) -> (36.5965, 7.9143) centre (33.4441, 15.267) ccw
  arc A133 (5.4488, -7.9563) -> (8.6206, -4.4287) centre (1.3533, -1.0841) ccw
  arc A134 (0.2433, 2.4112) -> (1.4026, 0.8155) centre (14.9574, 11.8827) ccw
  arc A135 (36.7638, 8.97) -> (32.4286, 10.8965) centre (31.4935, 2.9514) ccw
  arc A136 (-0.2164, -4.047) -> (3.8903, -1.6722) centre (-1.9878, 3.7545) ccw
  arc A137 (28.5123, 22.9498) -> (30.8871, 27.0565) centre (23.0856, 28.8279) ccw
  arc A138 (19.4184, -5.0382) -> (21.2942, -4.4287) centre (14.9574, 11.8827) ccw
  arc A139 (17.8701, -9.9237) -> (18.9258, -9.7564) centre (14.9574, 11.8827) ccw
  arc A140 (30.8871, -3.2912) -> (28.5123, 0.8155) centre (23.0856, -5.0625) ccw
  arc A141 (21.2942, 28.194) -> (19.4184, 28.8035) centre (14.9574, 11.8827) ccw
  arc A142 (36.5965, 15.8511) -> (31.8783, 16.3437) centre (33.4441, 8.4984) ccw
  arc A143 (-1.9634, 16.3437) -> (-6.6817, 15.8511) centre (-3.5292, 8.4984) ccw
  arc A144 (-6.8489, 14.7954) -> (-2.5138, 12.8689) centre (-1.5786, 20.814) ccw
  arc A145 (29.6716, 21.3542) -> (28.5123, 22.9498) centre (14.9574, 11.8827) ccw
  arc A146 (8.6206, -4.4287) -> (10.4964, -5.0382) centre (14.9574, 11.8827) ccw
  arc A147 (-4.8816, 21.3913) -> (-1.3539, 18.2195) centre (1.9907, 25.4868) ccw
  arc A148 (26.0246, 25.4375) -> (24.4289, 26.5968) centre (14.9574, 11.8827) ccw
  arc A149 (3.8903, 25.4375) -> (-0.2164, 27.8123) centre (-1.9878, 20.0109) ccw
  arc A150 (17.8701, 33.689) -> (15.9436, 29.3539) centre (23.8887, 28.4187) ccw
  arc A151 (-1.9634, 7.4217) -> (-1.3539, 5.5459) centre (14.9574, 11.8827) ccw
  arc A152 (15.9436, 29.3539) -> (13.9712, 29.3539) centre (14.9574, 11.8827) ccw
  arc A153 (31.8783, 16.3437) -> (31.2688, 18.2195) centre (14.9574, 11.8827) ccw
  arc A154 (-6.6817, 15.8511) -> (-6.8489, 14.7954) centre (14.9574, 11.8827) ccw
  arc A155 (-1.3539, 5.5459) -> (-4.8816, 2.374) centre (1.9907, -1.7214) ccw
  arc A156 (24.4661, 31.7217) -> (21.2942, 28.194) centre (28.5615, 24.8494) ccw
  arc A157 (-0.2164, 27.8123) -> (-0.9722, 27.0565) centre (14.9574, 11.8827) ccw
  arc A158 (31.2688, 18.2195) -> (34.7964, 21.3913) centre (27.9242, 25.4868) ccw
  arc A159 (31.2688, 5.5459) -> (31.8783, 7.4217) centre (14.9574, 11.8827) ccw
  circle A160 centre (14.9574, 11.8827) radius 2.75
  dimension "d4" = 5.5
  constraint concentric A145 A160
  measures "d4" diameter of A160
extrude "Extrude1" add sketch "Sketch1" along normal blind 6

design "Crank_B"
Autodesk Fusion 360 part; units mm, degrees
sketch "Sketch1" plane through (0, 0, 0) normal (0, 1, 0) x (1, 0, 0)
  arc A0 (12.5, 96.75) -> (-12.5, 96.75) centre (0, 96.75) ccw
  line L0 (12.5, 96.75) -> (12.5, 10.75)
  arc A1 (-12.5, 10.75) -> (12.5, 10.75) centre (0, 10.75) ccw
  circle A2 centre (0, 96.75) radius 3
  circle A3 centre (0, 10.75) radius 3
  line L1 (-12.5, 10.75) -> (-12.5, 96.75)
  constraint parallel L0 L1
  constraint concentric A1 A3
extrude "Extrude1" add sketch "Sketch1" along normal blind 6

design "stamp pad"
Autodesk Fusion 360 part; units mm, degrees
sketch "Sketch1" plane through (0, 0, 0) normal (1, 0, 0) x (0, 0, -1)
  line L0 (-50, 30) -> (50, 30)
  line L1 (50, 30) -> (50, -30)
  line L2 (50, -30) -> (-50, -30)
  line L3 (-50, -30) -> (-50, 30)
  line L4 (48, -28) -> (-48, -28)
  line L5 (-48, -28) -> (-48, 28)
  line L6 (-48, 28) -> (48, 28)
  line L7 (48, 28) -> (48, -28)
  dimension "d1" = 100
  dimension "d2" = 60
  dimension "d3" = 2
  dimension "d17" = 30
  dimension "d18" = 50
  constraint horizontal L0
  constraint perpendicular L0 L1
  constraint parallel L0 L2
  constraint parallel L1 L3
  measures "d1" distance of L1.end L2.end
  measures "d2" distance of L0.end L1.end
  measures "d17" distance of L0 origin
  measures "d18" distance of origin L3
extrude "Extrude1" add sketch "Sketch1" along normal blind 2 contours L0 L1 L2 L3 | L4 L5 L6 L7
extrude "Extrude2" add sketch "Sketch1" against normal blind 15
sketch "Sketch2" plane through (0, 0, 0) normal (-1, 0, 0) x (0, 0, 1)
  line L0 (-48, 28) -> (-48, -28)
  line L1 (-48, -28) -> (48, -28)
  line L2 (48, -28) -> (48, 28)
  line L3 (48, 28) -> (-48, 28)
  line L4 (45, 25) -> (-45, 25)
  line L5 (-45, 25) -> (-45, -25)
  line L6 (-45, -25) -> (45, -25)
  line L7 (45, -25) -> (45, 25)
  line L8 (45, 25) -> (-45, -25) construction
  line L9 (-45, 25) -> (45, -25) construction
  dimension "d8" = 90
  dimension "d9" = 50
  constraint horizontal L4
  constraint perpendicular L4 L5
  constraint parallel L4 L6
  constraint parallel L5 L7
  constraint coincident L8 origin
  constraint coincident L9 origin
  measures "d8" distance of L5.end L6.end
  measures "d9" distance of L4.end L5.end
extrude "Extrude3" add sketch "Sketch2" along normal blind 13 contours L4 L5 L6 L7
sketch "Sketch4" plane through (2, 0, 0) normal (1, 0, 0) x (0, 0, -1)
  line L0 (-50, -30) -> (50, -30)
  line L1 (50, -30) -> (50, 30)
  line L2 (50, 30) -> (-50, 30)
  line L3 (-50, 30) -> (-50, -30)
  line L4 (-50, 10) -> (150, 10)
  line L5 (150, 10) -> (150, -10)
  line L6 (150, -10) -> (-50, -10)
  line L7 (-50, -10) -> (-50, 10)
  constraint horizontal L4
  constraint vertical L5
  constraint horizontal L6
  constraint vertical L7
  constraint coincident L3 L4.start
extrude "Extrude4" add sketch "Sketch4" along normal blind 6 contours L1 L3 L4 L6 L7 | L1 L4 L5 L6
sketch "Sketch5" plane through (0, -10, 0) normal (0, -1, 0) x (1, 0, 0)
  line L0 (2, -50) -> (2, -150)
  line L1 (2, -150) -> (8, -150)
  line L2 (8, -150) -> (8, 50)
  line L3 (8, 50) -> (2, 50)
  line L4 (2, 50) -> (2, -50)
  line L5 (28, -115) -> (28, -85)
  line L6 (28, -85) -> (8, -85)
  arc A0 (8, -115) -> (28, -115) centre (18, -115) ccw
  circle A1 centre (18, -115) radius 3
  dimension "d28" = 6
  constraint vertical L5
  constraint coincident L2 L6.end
  constraint perpendicular L2 L6
  constraint coincident L2 A0.start
  constraint concentric A0 A1
  measures "d28" diameter of A1
extrude "Extrude5" add sketch "Sketch5" against normal blind 10 from surface at -5 contours L2 L5 L6 A0

design "rod2"
Autodesk Fusion 360 part; units mm, degrees
sketch "Sketch1" plane through (0, 0, 0) normal (1, 0, 0) x (0, 0, -1)
  circle A0 centre (0, 0) radius 3
  dimension "d1" = 6
  constraint coincident A0.centre origin
  measures "d1" diameter of A0
extrude "Extrude1" add sketch "Sketch1" along normal blind 45

design "stamp support"
Autodesk Fusion 360 part; units mm, degrees
sketch "Sketch1" plane through (0, 0, 0) normal (1, 0, 0) x (0, 0, -1)
  line L0 (-10, 140) -> (10, 140)
  line L1 (10, 140) -> (10, -140)
  line L2 (10, -140) -> (-10, -140)
  line L3 (-10, -140) -> (-10, 140)
  circle A0 centre (0, 130) radius 3
  dimension "d1" = 20
  dimension "d2" = 280
  dimension "d3" = 6
  dimension "d4" = 10
  constraint horizontal L0
  constraint perpendicular L0 L1
  constraint parallel L0 L2
  constraint parallel L1 L3
  measures "d1" distance of L1.end L2.end
  measures "d2" distance of L0.end L1.end
  measures "d3" diameter of A0
  measures "d4" distance of L0 A0.centre
extrude "Extrude1" add sketch "Sketch1" along normal blind 6

design "Rocker_B"
Autodesk Fusion 360 part; units mm, degrees
sketch "Sketch1" plane through (0, 0, 0) normal (0, 1, 0) x (1, 0, 0)
  circle A0 centre (0, 96.75) radius 3
  arc A1 (12.5, 96.75) -> (-12.5, 96.75) centre (0, 96.75) ccw
  line L0 (12.5, 96.75) -> (12.5, -53.25)
  arc A2 (-12.5, -53.25) -> (12.5, -53.25) centre (0, -53.25) ccw
  line L1 (-12.5, -53.25) -> (-12.5, 96.75)
  circle A3 centre (0, -53.25) radius 3
  point P0 (-35.6168, 0)
  constraint parallel L0 L1
  constraint concentric A2 A3
extrude "Extrude1" add sketch "Sketch1" along normal blind 6

design "support disk"
Autodesk Fusion 360 part; units mm, degrees
sketch "Sketch1" plane through (0, 0, 0) normal (1, 0, 0) x (0, 0, -1)
  circle A0 centre (0, 0) radius 3
  circle A1 centre (0, 0) radius 40
  dimension "d1" = 6
  dimension "d2" = 80
  constraint coincident A0.centre A1.centre
  measures "d1" diameter of A0
  measures "d2" diameter of A1
extrude "Extrude1" add sketch "Sketch1" along normal blind 6
